Meanwell LRS-350-24 Power Supply v2 (Autodesk Fusion 360 design; units mm, degrees)
Autodesk Fusion 360 part; units mm, degrees
sketch "Sketch1" plane through (0, 0, 0) normal (0, 0, 1) x (1, 0, 0)
  line L0 (0, 0) -> (215, 0)
  line L1 (215, 0) -> (215, 115)
  line L2 (215, 115) -> (0, 115)
  line L3 (0, 115) -> (0, 0)
  circle A0 centre (32.5, 32.5) radius 1.58
  circle A1 centre (32.5, 82.5) radius 1.58
  circle A2 centre (182.5, 82.5) radius 1.58
  circle A3 centre (182.5, 32.5) radius 1.58
  dimension "d1" = 215
  dimension "d2" = 115
  dimension "d3" = 3.16
  dimension "d4" = 3.16
  dimension "d5" = 3.16
  dimension "d6" = 3.16
  dimension "d7" = 32.5
  dimension "d8" = 32.5
  dimension "d9" = 32.5
  dimension "d10" = 32.5
  dimension "d11" = 150
  dimension "d12" = 150
  dimension "d13" = 50
  dimension "d14" = 32.5
  constraint horizontal L0
  constraint vertical L1
  constraint horizontal L2
  constraint vertical L3
  constraint coincident L0.start L3.end
  measures "d3" diameter of A0
  measures "d4" diameter of A1
  measures "d5" diameter of A2
  measures "d6" diameter of A3
extrude "Extrude1" add sketch "Sketch1" along normal blind 30
move_face "OffsetFaces1" offset 5 1 faces at (34.0721, 32.3427, 20)
delete_face "DeleteFace1" 1 faces at (31.7792, 81.094, 20)
delete_face "DeleteFace2" 1 faces at (183.3572, 83.8272, 20)
delete_face "DeleteFace3" 1 faces at (182.6965, 34.0677, 20)
extrude "Extrude2" cut sketch "Sketch1" along normal blind 6 contours A0 | A1 | A2 | A3
sketch "Sketch2" plane through (0, 0, 0) normal (0, -1, 0) x (1, 0, 0)
  line L0 (0, 0) -> (215, 0)
  line L1 (215, 0) -> (215, 30)
  line L2 (215, 30) -> (0, 30)
  line L3 (0, 30) -> (0, 0)
  circle A0 centre (32.5, 12.5) radius 1.58
  circle A1 centre (182.5, 12.5) radius 1.58
  dimension "d20" = 3.16
  dimension "d21" = 3.16
  dimension "d22" = 32.5
  dimension "d23" = 32.5
  dimension "d24" = 12.5
  dimension "d25" = 12.5
  measures "d20" diameter of A0
  measures "d21" diameter of A1
extrude "Extrude3" cut sketch "Sketch2" against normal blind 115 contours A0 | A1
sketch "Sketch3" plane through (0, 0, 30) normal (0, 0, 1) x (-1, 0, 0)
  line L0 (0, -115) -> (0, 0)
  line L1 (0, 0) -> (-215, 0)
  line L2 (-215, 0) -> (-215, -115)
  line L3 (-215, -115) -> (0, -115)
  line L4 (0, -112.5) -> (-18.7833, -112.5)
  line L5 (-18.7833, -112.5) -> (-18.7833, -2.5)
  line L6 (-18.7833, -2.5) -> (0, -2.5)
  line L7 (0, -2.5) -> (0, -112.5)
  dimension "d28" = 2.5
  dimension "d29" = 2.5
  constraint horizontal L4
  constraint vertical L5
  constraint horizontal L6
  constraint vertical L7
  constraint coincident L0 L1.start
extrude "Extrude4" cut sketch "Sketch3" against normal blind 27.7 contours L0 L4 L5 L6 L7
sketch "Sketch4" plane through (18.7833, 0, 0) normal (-1, 0, 0) x (0, -1, 0)
  line L0 (-2.5, 30) -> (-112.5, 30)
  line L1 (-112.5, 30) -> (-112.5, 2.3)
  line L2 (-112.5, 2.3) -> (-2.5, 2.3)
  line L3 (-2.5, 2.3) -> (-2.5, 30)
  line L4 (-112.5, 2.3) -> (-2.5, 2.3)
  line L5 (-2.5, 2.3) -> (-2.5, 28.5)
  line L6 (-2.5, 28.5) -> (-112.5, 28.5)
  line L7 (-112.5, 28.5) -> (-112.5, 2.3)
  dimension "d32" = 26.2
  constraint horizontal L4
  constraint vertical L5
  constraint horizontal L6
  constraint vertical L7
extrude "Extrude5" cut sketch "Sketch4" against normal blind 194.217 contours L1 L2 L3 L4 L5 L6 L7
sketch "Sketch5" plane through (0, 0, 30) normal (0, 0, 1) x (-1, 0, 0)
  line L0 (-18.7833, -2.5) -> (0, -2.5)
  line L1 (0, -2.5) -> (0, 0)
  line L2 (0, 0) -> (-215, 0)
  line L3 (-215, 0) -> (-215, -115)
  line L4 (-215, -115) -> (0, -115)
  line L5 (0, -115) -> (0, -112.5)
  line L6 (0, -112.5) -> (-18.7833, -112.5)
  line L7 (-18.7833, -112.5) -> (-18.7833, -2.5)
  circle A0 centre (-167.55, -78.3) radius 25
  dimension "d35" = 50
  dimension "d36" = 47.45
  dimension "d37" = 36.7
  measures "d35" diameter of A0
  measures "d36" distance of L1.end
  measures "d37" distance of L1.end
extrude "Extrude6" cut sketch "Sketch5" against normal blind 7.617 contours A0
fillet "Fillet1" radius 3 2 edges at (0, 1.25, 30) (0, 113.75, 30)
fillet "Fillet2" radius 3 2 edges at (107.5, 115, 0) (107.5, 0, 0)
fillet "Fillet3" radius 1.5 2 edges at (106.5002, 112.5, 2.3) (106.5002, 2.5, 2.3)
equation "d30 = -30.00 mm + 2.3 mm"
equation "d32 = 27.700 mm - 1.5 mm"
